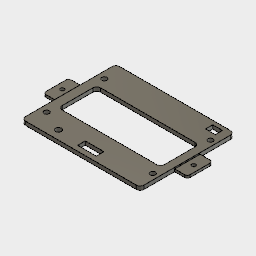
Support circuit lanterne - petit (Autodesk Fusion 360 design; units mm, degrees)
Autodesk Fusion 360 part; units mm, degrees
sketch "Sketch1" plane through (0, 0, 0) normal (0, 1, 0) x (1, 0, 0)
  circle A0 centre (18.4015, -12.4035) radius 2
  line L0 (-11, -35) -> (125, -35)
  line L1 (60, 10) -> (60, -83.0941)
  circle A1 centre (101.5985, -12.4035) radius 2
  circle A2 centre (18.4015, -57.5965) radius 2
  circle A3 centre (101.5985, -57.5965) radius 2
  line L2 (5, -45) -> (13, -45)
  line L3 (13, -45) -> (13, -25)
  line L4 (13, -25) -> (5, -25)
  line L5 (3, -27) -> (3, -43)
  circle A4 centre (8, -35) radius 1.5
  line L6 (97, -50) -> (23, -50)
  line L7 (20, -47) -> (20, -23)
  line L8 (23, -20) -> (97, -20)
  line L9 (100, -23) -> (100, -47)
  arc A5 (20, -47) -> (23, -50) centre (23, -47) ccw
  arc A6 (23, -20) -> (20, -23) centre (23, -23) ccw
  arc A7 (97, -50) -> (100, -47) centre (97, -47) ccw
  arc A8 (100, -23) -> (97, -20) centre (97, -23) ccw
  arc A9 (3, -43) -> (5, -45) centre (5, -43) ccw
  arc A10 (5, -25) -> (3, -27) centre (5, -27) ccw
  line L10 (106, -45) -> (114, -45)
  line L11 (116, -43) -> (116, -27)
  line L12 (114, -25) -> (106, -25)
  line L13 (106, -25) -> (106, -45)
  arc A11 (114, -45) -> (116, -43) centre (114, -43) ccw
  arc A12 (116, -27) -> (114, -25) centre (114, -27) ccw
  circle A13 centre (111, -35) radius 1.5
  line L14 (92.023, -6.7335) -> (99.623, -6.7335)
  line L15 (99.623, -6.7335) -> (99.623, -1.1335)
  line L16 (99.623, -1.1335) -> (92.023, -1.1335)
  line L17 (92.023, -1.1335) -> (92.023, -6.7335)
  circle A14 centre (35, -65) radius 2.25
  line L18 (53, -62) -> (67.6, -62)
  line L19 (67.6, -62) -> (67.6, -67.9)
  line L20 (67.6, -67.9) -> (53, -67.9)
  line L21 (53, -67.9) -> (53, -62)
  line L22 (13, -1) -> (13, -69)
  line L23 (16, -72) -> (103, -72)
  line L24 (106, -69) -> (106, -1)
  line L25 (103, 2) -> (16, 2)
  arc A15 (16, 2) -> (13, -1) centre (16, -1) ccw
  arc A16 (106, -1) -> (103, 2) centre (103, -1) ccw
  arc A17 (13, -69) -> (16, -72) centre (16, -69) ccw
  arc A18 (103, -72) -> (106, -69) centre (103, -69) ccw
  point P0 (0, -70)
  point P1 (3, -45)
  point P2 (116, -45)
  point P3 (109, -75)
  dimension "d8" = 4
  dimension "d11" = 10
  dimension "d12" = 3
  dimension "d17" = 3
  dimension "d18" = 3
  dimension "d19" = 3
  dimension "d20" = 3
  dimension "d21" = 2
  dimension "d22" = 2
  dimension "d33" = 10
  dimension "d34" = 2
  dimension "d35" = 2
  dimension "d36" = 3
  dimension "d51" = 7.6
  dimension "d52" = 5.6
  dimension "d53" = 4.5
  dimension "d54" = 5.9
  dimension "d55" = 14.6
  dimension "d63" = 3
  dimension "d64" = 3
  dimension "d65" = 3
  dimension "d66" = 3
  measures "d8" diameter of A0
  measures "d11" distance of P1 L2.end
  measures "d12" diameter of A4
  measures "d17" radius of A5
  measures "d18" radius of A6
  measures "d19" radius of A7
  measures "d20" radius of A8
  measures "d21" radius of A9
  measures "d22" radius of A10
  measures "d33" distance of L10.start P2
  measures "d34" radius of A11
  measures "d35" radius of A12
  measures "d36" diameter of A13
  measures "d51" distance of L14.start L14.end
  measures "d52" distance of L14.start L16.end
  measures "d53" diameter of A14
  measures "d54" distance of L18.start L20.end
  measures "d55" distance of L18.start L18.end
  measures "d63" radius of A15
  measures "d64" radius of A16
  measures "d65" radius of A17
  measures "d66" radius of A18
extrude "Extrude10" add sketch "Sketch1" along normal blind 3 contours L0 L1 L3 L7 L8 A6 L22 L25 A15 | L0 L1 L3 L6 L7 A5 L18 L20 L21 L22 L23 A17 | L0 L1 L8 L9 A8 L13 L24 L25 A16 | L0 L1 L6 L9 A7 L13 L18 L19 L20 L23 L24 A18
extrude "Extrude11" add sketch "Sketch1" along normal blind 2 contours L0 L3 L4 L5 A4 A10 L22 | L0 L2 L3 L5 A4 A9 L22 | L0 L11 L12 L13 A12 A13 L24 | L0 L10 L11 L13 A11 A13 L24
